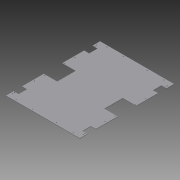
# Autodesk Inventor part: base
Saved by Autodesk Inventor 2015 SP1 (Build 190203100, 203)
## iProperties
Created: 2014-12-22
Part Number: base
Material: Generic
Document SubType Name: Modeling
Designer: Jarod
Density: 1 g/cm^3
Appearance: Default
Author: Jarod
Autodesk Inventor part; units mm, degrees
ref_plane "YZ Plane" through (0, 0, 0) normal (1, 0, 0) x (0, 1, 0)
ref_plane "XZ Plane" through (0, 0, 0) normal (0, 1, 0) x (-1, 0, 0)
ref_plane "XY Plane" through (0, 0, 0) normal (0, 0, 1) x (1, 0, 0)
sketch "Sketch1" plane through (0, 0, 0) normal (0, 1, 0) x (-1, 0, 0)
  line L0 (0, 0) -> (558.8, 0) construction
  line L1 (558.8, 0) -> (558.8, -711.2) construction
  line L2 (558.8, -711.2) -> (0, -711.2) construction
  line L3 (0, -711.2) -> (0, 0) construction
  line L4 (558.8, -355.6) -> (457.2, -355.6) construction
  line L5 (457.2, -355.6) -> (457.2, -425.45) construction
  line L6 (457.2, -425.45) -> (558.8, -425.45) construction
  line L7 (558.8, -425.45) -> (558.8, -355.6) construction
  line L8 (558.8, -355.6) -> (457.2, -355.6) construction
  line L9 (457.2, -355.6) -> (457.2, -285.75) construction
  line L10 (457.2, -285.75) -> (558.8, -285.75) construction
  line L11 (558.8, -285.75) -> (558.8, -355.6) construction
  line L12 (0, -355.6) -> (101.6, -355.6) construction
  line L13 (101.6, -355.6) -> (101.6, -425.45) construction
  line L14 (101.6, -425.45) -> (0, -425.45) construction
  line L15 (0, -425.45) -> (0, -355.6) construction
  line L16 (0, -355.6) -> (101.6, -355.6) construction
  line L17 (101.6, -355.6) -> (101.6, -285.75) construction
  line L18 (101.6, -285.75) -> (0, -285.75) construction
  line L19 (0, -285.75) -> (0, -355.6) construction
  line L20 (558.8, 0) -> (558.8, -57.15) construction
  line L21 (558.8, -57.15) -> (520.7, -57.15) construction
  line L22 (520.7, -57.15) -> (520.7, -120.65) construction
  line L23 (520.7, -120.65) -> (558.8, -120.65) construction
  line L24 (558.8, -120.65) -> (558.8, -57.15) construction
  line L25 (0, 0) -> (0, -57.15) construction
  line L26 (0, -57.15) -> (38.1, -57.15) construction
  line L27 (38.1, -57.15) -> (38.1, -120.65) construction
  line L28 (38.1, -120.65) -> (0, -120.65) construction
  line L29 (0, -120.65) -> (0, -57.15) construction
  line L30 (0, -711.2) -> (0, -654.05) construction
  line L31 (0, -654.05) -> (38.1, -654.05) construction
  line L32 (38.1, -654.05) -> (38.1, -590.55) construction
  line L33 (38.1, -590.55) -> (0, -590.55) construction
  line L34 (0, -590.55) -> (0, -654.05) construction
  line L35 (558.8, -711.2) -> (558.8, -654.05) construction
  line L36 (558.8, -654.05) -> (520.7, -654.05) construction
  line L37 (520.7, -654.05) -> (520.7, -590.55) construction
  line L38 (520.7, -590.55) -> (558.8, -590.55) construction
  line L39 (558.8, -590.55) -> (558.8, -654.05) construction
  line L40 (0, 0) -> (558.8, 0)
  line L41 (558.8, 0) -> (558.8, -57.15)
  line L42 (558.8, -57.15) -> (520.7, -57.15)
  line L43 (520.7, -57.15) -> (520.7, -120.65)
  line L44 (520.7, -120.65) -> (558.8, -120.65)
  line L45 (558.8, -120.65) -> (558.8, -285.75)
  line L46 (558.8, -285.75) -> (457.2, -285.75)
  line L47 (457.2, -285.75) -> (457.2, -425.45)
  line L48 (457.2, -425.45) -> (558.8, -425.45)
  line L49 (558.8, -425.45) -> (558.8, -590.55)
  line L50 (558.8, -590.55) -> (520.7, -590.55)
  line L51 (520.7, -590.55) -> (520.7, -654.05)
  line L52 (520.7, -654.05) -> (558.8, -654.05)
  line L53 (558.8, -654.05) -> (558.8, -711.2)
  line L54 (558.8, -711.2) -> (0, -711.2)
  line L55 (0, -711.2) -> (0, -654.05)
  line L56 (0, -654.05) -> (38.1, -654.05)
  line L57 (38.1, -654.05) -> (38.1, -590.55)
  line L58 (38.1, -590.55) -> (0, -590.55)
  line L59 (0, -590.55) -> (0, -425.45)
  line L60 (0, -425.45) -> (101.6, -425.45)
  line L61 (101.6, -425.45) -> (101.6, -285.75)
  line L62 (101.6, -285.75) -> (0, -285.75)
  line L63 (0, -285.75) -> (0, -120.65)
  line L64 (0, -120.65) -> (38.1, -120.65)
  line L65 (38.1, -120.65) -> (38.1, -57.15)
  line L66 (38.1, -57.15) -> (0, -57.15)
  line L67 (0, -57.15) -> (0, 0)
  dimension "d0" = 558.8
  dimension "d1" = 711.2
  dimension "d2" = 101.6
  dimension "d3" = 69.85
  dimension "d4" = 101.6
  dimension "d5" = 69.85
  dimension "d6" = 101.6
  dimension "d7" = 69.85
  dimension "d8" = 101.6
  dimension "d9" = 69.85
  dimension "d10" = 57.15
  dimension "d11" = 38.1
  dimension "d12" = 63.5
  dimension "d13" = 57.15
  dimension "d14" = 38.1
  dimension "d15" = 63.5
  dimension "d16" = 57.15
  dimension "d17" = 38.1
  dimension "d18" = 63.5
  dimension "d19" = 57.15
  dimension "d20" = 38.1
  dimension "d21" = 63.5
  constraints: 136 end point, 23 perpendicular, 18 parallel, 11 collinear, 9 horizontal, 4 point on line, 2 midpoint
  measures "d0" distance of L1.end L2.end
  measures "d1" distance of L0.end L1.end
  measures "d2" distance of L6.end L5.end
  measures "d3" distance of L5.end L4.end
  measures "d4" distance of L9.end L10.end
  measures "d5" distance of L8.end L9.end
  measures "d6" distance of L13.end L14.end
  measures "d7" distance of L12.end L13.end
  measures "d8" distance of L18.end L17.end
  measures "d9" distance of L17.end L16.end
  measures "d10" distance of L0.end L20.end
  measures "d11" distance of L23.end L22.end
  measures "d12" distance of L22.end L21.end
  measures "d13" distance of L0.start L25.end
  measures "d14" distance of L27.end L28.end
  measures "d15" distance of L26.end L27.end
  measures "d16" distance of L2.end L30.end
  measures "d17" distance of L33.end L32.end
  measures "d18" distance of L32.end L31.end
  measures "d19" distance of L1.end L35.end
  measures "d20" distance of L37.end L38.end
  measures "d21" distance of L36.end L37.end
extrude "Extrusion1" add sketch "Sketch1" along normal blind 3.175
sketch "Sketch2" plane through (0, 3.175, 0) normal (0, 1, 0) x (1, 0, 0)
  line L0 (-558.8, 0) -> (0, 0) projected
  line L1 (0, 0) -> (0, 57.15) projected
  line L2 (0, 57.15) -> (-38.1, 57.15) projected
  line L3 (-38.1, 57.15) -> (-38.1, 120.65) projected
  line L4 (-38.1, 120.65) -> (0, 120.65) projected
  line L5 (0, 120.65) -> (0, 285.75) projected
  line L6 (0, 285.75) -> (-101.6, 285.75) projected
  line L7 (-101.6, 285.75) -> (-101.6, 425.45) projected
  line L8 (-101.6, 425.45) -> (0, 425.45) projected
  line L9 (0, 425.45) -> (0, 590.55) projected
  line L10 (0, 590.55) -> (-38.1, 590.55) projected
  line L11 (-38.1, 590.55) -> (-38.1, 654.05) projected
  line L12 (-38.1, 654.05) -> (0, 654.05) projected
  line L13 (0, 654.05) -> (0, 711.2) projected
  line L14 (0, 711.2) -> (-558.8, 711.2) projected
  line L15 (-558.8, 711.2) -> (-558.8, 654.05) projected
  line L16 (-558.8, 654.05) -> (-520.7, 654.05) projected
  line L17 (-520.7, 654.05) -> (-520.7, 590.55) projected
  line L18 (-520.7, 590.55) -> (-558.8, 590.55) projected
  line L19 (-558.8, 590.55) -> (-558.8, 425.45) projected
  line L20 (-558.8, 425.45) -> (-457.2, 425.45) projected
  line L21 (-457.2, 425.45) -> (-457.2, 285.75) projected
  line L22 (-457.2, 285.75) -> (-558.8, 285.75) projected
  line L23 (-558.8, 285.75) -> (-558.8, 120.65) projected
  line L24 (-558.8, 120.65) -> (-520.7, 120.65) projected
  line L25 (-520.7, 120.65) -> (-520.7, 57.15) projected
  line L26 (-520.7, 57.15) -> (-558.8, 57.15) projected
  line L27 (-558.8, 57.15) -> (-558.8, 0) projected
  point P0 (-546.1, 38.1)
  point P1 (-546.1, 50.8)
  point P2 (-12.7, 38.1)
  point P3 (-12.7, 50.8)
  point P4 (-12.7, 673.1)
  point P5 (-12.7, 660.4)
  point P6 (-546.1, 673.1)
  point P7 (-546.1, 660.4)
  dimension "d24" = 12.7
  dimension "d25" = 12.7
  dimension "d26" = 50.8
  dimension "d27" = 38.1
  dimension "d28" = 12.7
  dimension "d29" = 12.7
  dimension "d30" = 38.1
  dimension "d31" = 50.8
  dimension "d32" = 50.8
  dimension "d33" = 38.1
  dimension "d34" = 38.1
  dimension "d35" = 50.8
  dimension "d36" = 12.7
  dimension "d37" = 12.7
  dimension "d38" = 12.7
  dimension "d39" = 12.7
  measures "d24" distance from line of L27 point (-546.1, 38.1)
  measures "d25" distance from line of L27 point (-546.1, 50.8)
  measures "d26" distance from line of L0 point (-546.1, 50.8)
  measures "d27" distance from line of L0 point (-546.1, 38.1)
  measures "d28" distance from line of L1 point (-12.7, 50.8)
  measures "d29" distance from line of L1 point (-12.7, 38.1)
  measures "d30" distance from line of L0 point (-12.7, 38.1)
  measures "d31" distance from line of L0 point (-12.7, 50.8)
  measures "d32" distance from line of L14 point (-12.7, 660.4)
  measures "d33" distance from line of L14 point (-12.7, 673.1)
  measures "d34" distance from line of L14 point (-546.1, 673.1)
  measures "d35" distance from line of L14 point (-546.1, 660.4)
  measures "d36" distance from line of L15 point (-546.1, 660.4)
  measures "d37" distance from line of L15 point (-546.1, 673.1)
  measures "d38" distance from line of L13 point (-12.7, 673.1)
  measures "d39" distance from line of L13 point (-12.7, 660.4)
hole "Hole1" at (-546.1, 3.175, -38.1) at (-546.1, 3.175, -50.8) at (-12.7, 3.175, -38.1) at (-12.7, 3.175, -50.8) at (-12.7, 3.175, -673.1) at (-12.7, 3.175, -660.4) at (-546.1, 3.175, -673.1) at (-546.1, 3.175, -660.4) direction (0, -1, 0) diameter 6.35 end through all
sketch "Sketch3" plane through (0, 0, 0) normal (0, -1, 0) x (1, 0, 0)
  circle A0 centre (-546.1, -673.1) radius 3.175 projected
  circle A1 centre (-12.7, -673.1) radius 3.175 projected
  circle A2 centre (-12.7, -38.1) radius 3.175 projected
  circle A3 centre (-546.1, -38.1) radius 3.175 projected
  circle A4 centre (-546.1, -50.8) radius 3.175 projected
  circle A5 centre (-12.7, -50.8) radius 3.175 projected
  circle A6 centre (-12.7, -660.4) radius 3.175 projected
  circle A7 centre (-546.1, -660.4) radius 3.175 projected
  line L0 (0, 0) -> (-558.8, 0) projected
  line L1 (-558.8, 0) -> (-558.8, -57.15) projected
  line L2 (-558.8, -57.15) -> (-520.7, -57.15) projected
  line L3 (-520.7, -57.15) -> (-520.7, -120.65) projected
  line L4 (-520.7, -120.65) -> (-558.8, -120.65) projected
  line L5 (-558.8, -120.65) -> (-558.8, -285.75) projected
  line L6 (-558.8, -285.75) -> (-457.2, -285.75) projected
  line L7 (-457.2, -285.75) -> (-457.2, -425.45) projected
  line L8 (-457.2, -425.45) -> (-558.8, -425.45) projected
  line L9 (-558.8, -425.45) -> (-558.8, -590.55) projected
  line L10 (-558.8, -590.55) -> (-520.7, -590.55) projected
  line L11 (-520.7, -590.55) -> (-520.7, -654.05) projected
  line L12 (-520.7, -654.05) -> (-558.8, -654.05) projected
  line L13 (-558.8, -654.05) -> (-558.8, -711.2) projected
  line L14 (-558.8, -711.2) -> (0, -711.2) projected
  line L15 (0, -711.2) -> (0, -654.05) projected
  line L16 (0, -654.05) -> (-38.1, -654.05) projected
  line L17 (-38.1, -654.05) -> (-38.1, -590.55) projected
  line L18 (-38.1, -590.55) -> (0, -590.55) projected
  line L19 (0, -590.55) -> (0, -425.45) projected
  line L20 (0, -425.45) -> (-101.6, -425.45) projected
  line L21 (-101.6, -425.45) -> (-101.6, -285.75) projected
  line L22 (-101.6, -285.75) -> (0, -285.75) projected
  line L23 (0, -285.75) -> (0, -120.65) projected
  line L24 (0, -120.65) -> (-38.1, -120.65) projected
  line L25 (-38.1, -120.65) -> (-38.1, -57.15) projected
  line L26 (-38.1, -57.15) -> (0, -57.15) projected
  line L27 (0, -57.15) -> (0, 0) projected
  point P0 (-12.7, -279.4)
  point P1 (-12.7, -203.2)
  point P2 (-12.7, -431.8)
  point P3 (-12.7, -508)
  point P4 (-546.1, -431.8)
  point P5 (-546.1, -508)
  point P6 (-546.1, -279.4)
  point P7 (-546.1, -203.2)
  dimension "d47" = 12.7
  dimension "d48" = 12.7
  dimension "d49" = 82.55
  dimension "d50" = 6.35
  dimension "d51" = 6.35
  dimension "d52" = 82.55
  dimension "d53" = 12.7
  dimension "d54" = 12.7
  dimension "d55" = 12.7
  dimension "d56" = 12.7
  dimension "d57" = 6.35
  dimension "d58" = 82.55
  dimension "d59" = 6.35
  dimension "d60" = 12.7
  dimension "d61" = 82.55
  dimension "d62" = 12.7
  measures "d47" distance from line of L5 point (-546.1, -279.4)
  measures "d48" distance from line of L5 point (-546.1, -203.2)
  measures "d49" distance from line of L6 point (-546.1, -203.2)
  measures "d50" distance from line of L6 point (-546.1, -279.4)
  measures "d51" distance from line of point (-546.1, -431.8) L8
  measures "d52" distance from line of point (-546.1, -508) L8
  measures "d53" distance from line of L9 point (-546.1, -508)
  measures "d54" distance from line of L9 point (-546.1, -431.8)
  measures "d55" distance from line of L23 point (-12.7, -279.4)
  measures "d56" distance from line of L23 point (-12.7, -203.2)
  measures "d57" distance from line of L22 point (-12.7, -279.4)
  measures "d58" distance from line of point (-12.7, -203.2) L22
  measures "d59" distance from line of L20 point (-12.7, -431.8)
  measures "d60" distance from line of point (-12.7, -431.8) L19
  measures "d61" distance from line of L20 point (-12.7, -508)
  measures "d62" distance from line of L19 point (-12.7, -508)
hole "Hole2" at (-12.7, 0, -279.4) at (-12.7, 0, -203.2) at (-12.7, 0, -431.8) at (-12.7, 0, -508) at (-546.1, 0, -431.8) at (-546.1, 0, -508) at (-546.1, 0, -279.4) at (-546.1, 0, -203.2) direction (0, 1, 0) diameter 6.35 end through all
sketch "Sketch4" plane through (0, 0, 0) normal (0, -1, 0) x (1, 0, 0)
  circle A0 centre (-546.1, -279.4) radius 3.175 projected
  circle A1 centre (-546.1, -431.8) radius 3.175 projected
  circle A2 centre (-12.7, -431.8) radius 3.175 projected
  circle A3 centre (-12.7, -279.4) radius 3.175 projected
  circle A4 centre (-12.7, -203.2) radius 3.175 projected
  circle A5 centre (-12.7, -508) radius 3.175 projected
  circle A6 centre (-546.1, -508) radius 3.175 projected
  circle A7 centre (-546.1, -203.2) radius 3.175 projected
  circle A8 centre (-546.1, -673.1) radius 3.175 projected
  circle A9 centre (-12.7, -673.1) radius 3.175 projected
  circle A10 centre (-12.7, -38.1) radius 3.175 projected
  circle A11 centre (-546.1, -38.1) radius 3.175 projected
  circle A12 centre (-546.1, -50.8) radius 3.175 projected
  circle A13 centre (-12.7, -50.8) radius 3.175 projected
  circle A14 centre (-12.7, -660.4) radius 3.175 projected
  circle A15 centre (-546.1, -660.4) radius 3.175 projected
  line L0 (0, 0) -> (-558.8, 0) projected
  line L1 (-558.8, 0) -> (-558.8, -57.15) projected
  line L2 (-558.8, -57.15) -> (-520.7, -57.15) projected
  line L3 (-520.7, -57.15) -> (-520.7, -120.65) projected
  line L4 (-520.7, -120.65) -> (-558.8, -120.65) projected
  line L5 (-558.8, -120.65) -> (-558.8, -285.75) projected
  line L6 (-558.8, -285.75) -> (-457.2, -285.75) projected
  line L7 (-457.2, -285.75) -> (-457.2, -425.45) projected
  line L8 (-457.2, -425.45) -> (-558.8, -425.45) projected
  line L9 (-558.8, -425.45) -> (-558.8, -590.55) projected
  line L10 (-558.8, -590.55) -> (-520.7, -590.55) projected
  line L11 (-520.7, -590.55) -> (-520.7, -654.05) projected
  line L12 (-520.7, -654.05) -> (-558.8, -654.05) projected
  line L13 (-558.8, -654.05) -> (-558.8, -711.2) projected
  line L14 (-558.8, -711.2) -> (0, -711.2) projected
  line L15 (0, -711.2) -> (0, -654.05) projected
  line L16 (0, -654.05) -> (-38.1, -654.05) projected
  line L17 (-38.1, -654.05) -> (-38.1, -590.55) projected
  line L18 (-38.1, -590.55) -> (0, -590.55) projected
  line L19 (0, -590.55) -> (0, -425.45) projected
  line L20 (0, -425.45) -> (-101.6, -425.45) projected
  line L21 (-101.6, -425.45) -> (-101.6, -285.75) projected
  line L22 (-101.6, -285.75) -> (0, -285.75) projected
  line L23 (0, -285.75) -> (0, -120.65) projected
  line L24 (0, -120.65) -> (-38.1, -120.65) projected
  line L25 (-38.1, -120.65) -> (-38.1, -57.15) projected
  line L26 (-38.1, -57.15) -> (0, -57.15) projected
  line L27 (0, -57.15) -> (0, 0) projected
  point P0 (-495.3, -698.5)
  point P1 (-368.3, -698.5)
  point P2 (-190.5, -698.5)
  point P3 (-63.5, -698.5)
  point P4 (-495.3, -12.7)
  point P5 (-368.3, -12.7)
  point P6 (-190.5, -12.7)
  point P7 (-63.5, -12.7)
  dimension "d70" = 63.5
  dimension "d71" = 12.7
  dimension "d72" = 12.7
  dimension "d73" = 190.5
  dimension "d74" = 63.5
  dimension "d75" = 12.7
  dimension "d76" = 12.7
  dimension "d77" = 190.5
  dimension "d78" = 12.7
  dimension "d79" = 63.5
  dimension "d80" = 12.7
  dimension "d81" = 190.5
  dimension "d82" = 63.5
  dimension "d83" = 12.7
  dimension "d84" = 12.7
  dimension "d85" = 190.5
  measures "d70" distance from line of L15 point (-63.5, -698.5)
  measures "d71" distance from line of L14 point (-63.5, -698.5)
  measures "d72" distance from line of L14 point (-190.5, -698.5)
  measures "d73" distance from line of L15 point (-190.5, -698.5)
  measures "d74" distance from line of point (-495.3, -698.5) L13
  measures "d75" distance from line of L14 point (-495.3, -698.5)
  measures "d76" distance from line of L14 point (-368.3, -698.5)
  measures "d77" distance from line of L13 point (-368.3, -698.5)
  measures "d78" distance from line of L0 point (-495.3, -12.7)
  measures "d79" distance from line of L1 point (-495.3, -12.7)
  measures "d80" distance from line of L0 point (-368.3, -12.7)
  measures "d81" distance from line of point (-368.3, -12.7) L1
  measures "d82" distance from line of point (-63.5, -12.7) L27
  measures "d83" distance from line of L0 point (-63.5, -12.7)
  measures "d84" distance from line of L0 point (-190.5, -12.7)
  measures "d85" distance from line of point (-190.5, -12.7) L27
hole "Hole3" at (-495.3, 0, -698.5) at (-368.3, 0, -698.5) at (-190.5, 0, -698.5) at (-63.5, 0, -698.5) at (-495.3, 0, -12.7) at (-368.3, 0, -12.7) at (-190.5, 0, -12.7) at (-63.5, 0, -12.7) direction (0, 1, 0) diameter 6.35 end through all
body "Solid1"
